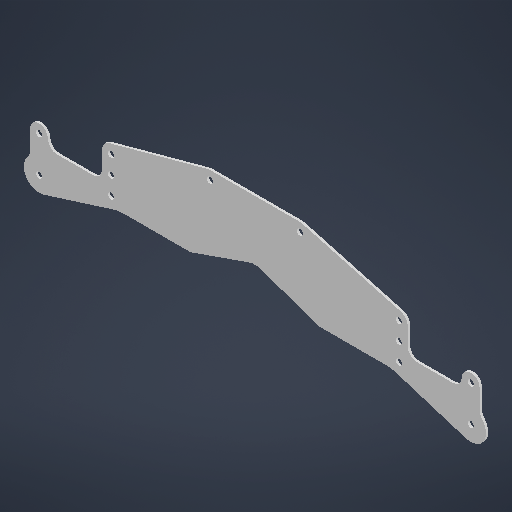
# Autodesk Inventor part: backaligner
Saved by Autodesk Inventor 2025.2 (Build 292293000, 293)
## iProperties
Created: 2025-01-15
Part Number: backaligner
Material: Generic
Document SubType Name: Modeling
Designer: Jahan
Density: 1 g/cm^3
Appearance: Default
Author: Jahan
Autodesk Inventor part; units mm, degrees
ref_plane "YZ Plane" through (0, 0, 0) normal (1, 0, 0) x (0, 1, 0)
ref_plane "XZ Plane" through (0, 0, 0) normal (0, 1, 0) x (-1, 0, 0)
ref_plane "XY Plane" through (0, 0, 0) normal (0, 0, 1) x (1, 0, 0)
sketch "Sketch1" plane through (0, 0, 0) normal (0, 0, 1) x (1, 0, 0)
  arc A0 (155.049, 9.8568) -> (142.3409, 9.8568) centre (148.6949, 9.8608) ccw
  circle A1 centre (148.6949, 9.8568) radius 2.1844
  circle A2 centre (148.6949, -15.5432) radius 2.1844
  line L0 (155.049, -4.0298) -> (155.049, 9.8568)
  arc A3 (155.049, -4.0298) -> (156.6938, -8.2941) centre (161.399, -4.0298) ccw
  arc A4 (145.4545, -25.8404) -> (156.6938, -8.2941) centre (148.6949, -15.5432) ccw
  arc A5 (135.9949, 3.5068) -> (142.3409, 9.8568) centre (135.9949, 9.8527) ccw
  line L1 (135.9949, 3.5068) -> (110.5949, 3.5068)
  arc A6 (104.2449, 9.8568) -> (110.5949, 3.5068) centre (110.5949, 9.8568) ccw
  line L2 (104.2449, 9.8568) -> (104.2449, 22.5568)
  circle A7 centre (97.8949, 9.8568) radius 2.1844
  circle A8 centre (97.8949, -2.8432) radius 2.1844
  circle A9 centre (97.8949, 22.5568) radius 2.1844
  circle A10 centre (-105.3051, 9.8568) radius 2.1844
  circle A11 centre (-105.3051, -2.8432) radius 2.1844
  circle A12 centre (-105.3051, 22.5568) radius 2.1844
  circle A13 centre (-156.1051, 9.8568) radius 2.1844
  circle A14 centre (-156.1051, -15.5432) radius 2.1844
  arc A15 (-164.1039, -8.2941) -> (-152.8646, -25.8404) centre (-156.1051, -15.5432) ccw
  line L3 (-162.4591, -4.0298) -> (-162.4591, 9.8568)
  arc A16 (-164.1039, -8.2941) -> (-162.4591, -4.0298) centre (-168.8091, -4.0298) ccw
  arc A17 (-149.751, 9.8568) -> (-162.4591, 9.8568) centre (-156.1051, 9.8608) ccw
  arc A18 (-149.751, 9.8568) -> (-143.4051, 3.5068) centre (-143.4051, 9.8527) ccw
  line L4 (-143.4051, 3.5068) -> (-118.0051, 3.5068)
  arc A19 (-118.0051, 3.5068) -> (-111.6551, 9.8568) centre (-118.0051, 9.8568) ccw
  line L5 (-111.6551, 9.8568) -> (-111.6551, 22.5568)
  circle A20 centre (-35.4551, 41.6068) radius 2.1844
  circle A21 centre (28.0449, 41.6068) radius 2.1844
  line L6 (-35.4551, 47.9568) -> (28.0449, 47.9568)
  line L7 (99.506, 28.699) -> (29.7157, 47.733)
  arc A22 (0.4819, 5.2197) -> (-7.892, 5.2197) centre (-3.7051, -6.7703) ccw
  arc A23 (40.7475, -8.8412) -> (42.841, -9.1962) centre (42.841, -2.8462) ccw
  line L8 (40.7475, -8.8412) -> (0.4819, 5.2197)
  arc A24 (-50.2511, -9.1962) -> (-48.1577, -8.8412) centre (-50.2511, -2.8462) ccw
  line L9 (-7.892, 5.2197) -> (-48.1577, -8.8412)
  arc A25 (104.2449, 22.5568) -> (99.506, 28.699) centre (97.8949, 22.5568) ccw
  line L10 (-106.9759, 28.683) -> (-37.1259, 47.733)
  arc A26 (-35.4551, 47.9568) -> (-37.1259, 47.733) centre (-35.4551, 41.6068) ccw
  arc A27 (29.7157, 47.733) -> (28.0449, 47.9568) centre (28.0449, 41.6068) ccw
  arc A28 (-106.9759, 28.683) -> (-111.6551, 22.5568) centre (-105.3051, 22.5568) ccw
  arc A29 (-96.072, -9.1962) -> (-103.6966, -10.3676) centre (-96.072, -34.5962) ccw
  arc A30 (96.2864, -10.3676) -> (88.6619, -9.1962) centre (88.6619, -34.5962) ccw
  line L11 (-103.6966, -10.3676) -> (-152.8646, -25.8404)
  line L12 (-96.072, -9.1962) -> (-50.2511, -9.1962)
  line L13 (88.6619, -9.1962) -> (42.841, -9.1962)
  line L14 (96.2864, -10.3676) -> (145.4545, -25.8404)
  point P0 (0, 0)
  dimension "d0" = 12.7
  dimension "d1" = 6.35
  dimension "d2" = 6.35
  dimension "d3" = 25.4
  dimension "d4" = 25.4
  constraints: 40 point on circle, 31 centre point, 30 end point, 4 coincident, 2 horizontal, 1 tangent
  measures "d0" radius of A22
  measures "d1" radius of A23
  measures "d2" radius of A24
  measures "d3" radius of A29
  measures "d4" radius of A30
extrude "Extrusion1" add sketch "Sketch1" along normal blind 1.5875
body "Solid1"
